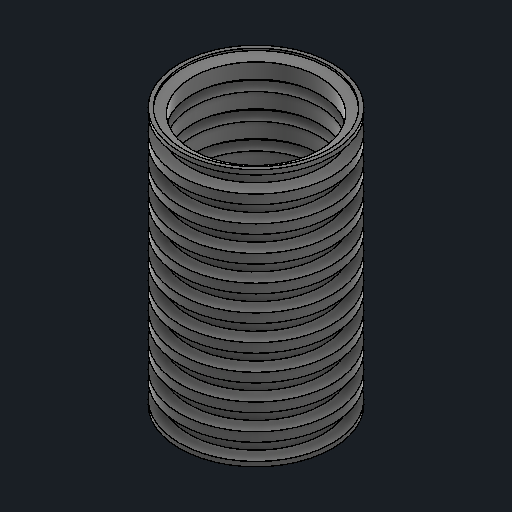
# Autodesk Inventor part: 40mm Vacuum Hose
Saved by Autodesk Inventor 2026.2 (Build 302298000, 298)
## iProperties
Created: 2026-07-12
Part Number: 40mm Vacuum Hose
Material: PVC, Unplasticized
Document SubType Name: Modeling
Designer: JoshuaEah
Density: 1.29 g/cm^3
Appearance: Smooth - Black
Author: JoshuaEah
Autodesk Inventor part; units mm, degrees
ref_plane "YZ Plane" through (0, 0, 0) normal (1, 0, 0) x (0, 1, 0)
ref_plane "XZ Plane" through (0, 0, 0) normal (0, 1, 0) x (-1, 0, 0)
ref_plane "XY Plane" through (0, 0, 0) normal (0, 0, 1) x (1, 0, 0)
sketch "Sketch2" plane through (0, 0, 0) normal (0, 0, 1) x (1, 0, 0)
  line L0 (0, 0) -> (20.75, 0)
  line L1 (0, 3.5) -> (18.25, 3.5)
  line L2 (20.75, 1.25) -> (20.75, 0)
  line L3 (0, 0) -> (0, 3.5)
  line L4 (18.25, 3.5) -> (18.25, 2.1599)
  line L5 (17.25, 3.5) -> (17.25, 1.4597)
  line L6 (19.75, 0) -> (19.75, 0.5498)
  line L7 (19.75, 0.5498) -> (17.25, 1.4597)
  line L8 (20.75, 1.25) -> (18.25, 2.1599)
  dimension "d4" = 1.25
  dimension "d6" = 36.5
  dimension "d7" = 41.5
  dimension "d9" = 34.5
  dimension "d10" = 1
  dimension "d12" = 1
  dimension "d15" = 110
  dimension "d16" = 1
  dimension "d17" = 2.25
  constraints: 19 end point, 3 vertical, 2 horizontal, 2 point on line, 1 coincident, 1 parallel, 1 perpendicular
  measures "d4" distance of L2.start L0.end
  measures "d6" diameter of L4 L3
  measures "d7" diameter of L2 L3
  measures "d9" diameter of L5 L3
  measures "d10" distance between parallel lines of L4 L5
  measures "d12" distance between parallel lines of L2 L6
  measures "d15" angle of L4 L8
  measures "d16" distance between parallel lines of L8 L7
  measures "d17" distance from line of L1 L2.start
revolve "Revolution1" add sketch "Sketch2" angle 360 about axis through (0, 0, 0) along (0, 1, 0) contours L6 L7 L5 L1 L4 L8 L2 L0
mirror "Mirror1" about plane through (17.25, 3.5, 0) normal (0, 1, 0) of "Revolution1"
pattern_linear "Rectangular Pattern1" count 10 spacing 7 along (0, 1, 0) of "Revolution1", "Mirror1"
equation "\"d12\" = d10"
equation "\"d16\" = d10"
body "Solid1"
